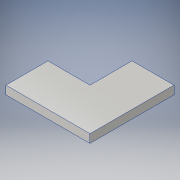
# Autodesk Inventor part: Angle Bracket
Saved by Autodesk Inventor 2016 (Build 200138000, 138)
## iProperties
Created: 2018-05-16
Part Number: Angle Bracket
Material: Aluminum 6061
Document SubType Name: Modeling
Designer: Kade
Density: 2.7 g/cm^3
Appearance: Aluminum - Flat
Author: Kade
Autodesk Inventor part; units mm, degrees
ref_plane "YZ Plane" through (0, 0, 0) normal (1, 0, 0) x (0, 1, 0)
ref_plane "XZ Plane" through (0, 0, 0) normal (0, 1, 0) x (-1, 0, 0)
ref_plane "XY Plane" through (0, 0, 0) normal (0, 0, 1) x (1, 0, 0)
sketch "Sketch1" plane through (0, 0, 0) normal (0, 1, 0) x (-1, 0, 0)
  line L0 (0, 0) -> (6.35, 0)
  line L1 (6.35, 0) -> (6.35, -3.175)
  line L2 (6.35, -3.175) -> (3.175, -3.175)
  line L3 (3.175, -3.175) -> (3.175, -6.35)
  line L4 (3.175, -6.35) -> (0, -6.35)
  line L5 (0, -6.35) -> (0, 0)
  dimension "d0" = 6.35
  dimension "d1" = 3.175
  dimension "d2" = 90
  dimension "d3" = 3.175
  dimension "d4" = 3.175
  constraints: 12 end point, 2 horizontal, 2 perpendicular, 1 vertical
  measures "d0" distance of L0.start L0.end
  measures "d1" distance of L0.end L1.end
  measures "d2" angle of L0 L1
  measures "d3" distance of L1.end L2.end
  measures "d4" distance of L2.end L3.end
extrude "Extrusion1" add sketch "Sketch1" along normal blind 0.635
body "Solid1"
